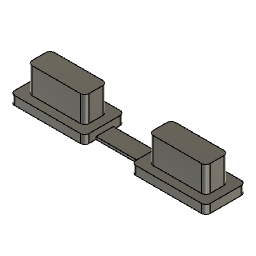
Button Cap (Autodesk Fusion 360 design; units mm, degrees)
Autodesk Fusion 360 part; units mm, degrees
sketch "草图1" plane through (0, 0, 0) normal (0, 0, 1) x (1, 0, 0)
  line L0 (20.6, 0) -> (20.6, -2.6)
  line L1 (0, -2.6) -> (0, 0)
  line L2 (6.6, 0) -> (6.6, -2.6)
  line L3 (14, 0) -> (14, -2.6)
  line L4 (0, 0) -> (6.6, 0)
  line L5 (14, 0) -> (20.6, 0)
  line L6 (20.6, -2.6) -> (14, -2.6)
  line L7 (6.6, -2.6) -> (0, -2.6)
  line L8 (7.6, -3.6) -> (-1, -3.6)
  line L9 (-1, -3.6) -> (-1, 1)
  line L10 (-1, 1) -> (7.6, 1)
  line L11 (7.6, 1) -> (7.6, -3.6)
  line L12 (21.6, -3.6) -> (13, -3.6)
  line L13 (13, 1) -> (13, -3.6)
  line L14 (13, 1) -> (21.6, 1)
  line L15 (21.6, 1) -> (21.6, -3.6)
  line L16 (7.6, -0.3) -> (13, -0.3)
  line L17 (7.6, -2.3) -> (13, -2.3)
  dimension "d2" = 2.6
  dimension "d3" = 6.6
  dimension "d4" = 6.6
  dimension "d7" = -1
  dimension "d8" = -1
  dimension "d9" = 2
  dimension "d10" = 0.3
  dimension "d19" = 5.4
  constraint horizontal L4
  constraint vertical L0
  constraint horizontal L6
  constraint vertical L1
  constraint coincident L1.end L4.start
  constraint coincident L2.end L6
  constraint perpendicular L2 L6
  constraint coincident L3.start L4
  constraint perpendicular L3 L6
  constraint collinear L4 L5
  constraint collinear L6 L7
  constraint coincident L11 L16.start
  constraint coincident L13 L16.end
  constraint perpendicular L13 L16
  constraint coincident L11 L17.start
  constraint coincident L13 L17.end
  constraint perpendicular L13 L17
  measures "d2" distance of L1.end L1.start
  measures "d3" distance of L1 L2
  measures "d4" distance of L0 L3
  measures "d9" distance of L16 L17
  measures "d10" distance of L4 L16
  measures "d19" distance of L16.start L16.end
extrude "拉伸1" add sketch "草图1" along normal blind 1 contours L0 L3 L5 L6 | L1 L2 L4 L7 | L8 L9 L10 L11 | L12 L13 L14 L15 makes body 1 at (1.8667, -0.5333, 0) makes body 2 at (18.7333, -2.0667, 0)
extrude "拉伸2" add sketch "草图1" along normal blind 0.3 contours L11 L13 L16 L17 bodies 1 2
extrude "拉伸3" add sketch "草图1" along normal blind 4 contours L0 L3 L5 L6 | L1 L2 L4 L7 bodies 1
fillet "圆角1" radius 0.5 16 edges at (6.6, -2.6, 2.5) (6.6, 0, 2.5) (0, 0, 2.5) (0, -2.6, 2.5) (-1, -3.6, 0.5) (-1, 1, 0.5) (7.6, 1, 0.5) (7.6, -3.6, 0.5) (14, -2.6, 2.5) (13, -3.6, 0.5) (13, 1, 0.5) (21.6, -3.6, 0.5) (21.6, 1, 0.5) (20.6, 0, 2.5) (20.6, -2.6, 2.5) (14, 0, 2.5) on bodies 1
